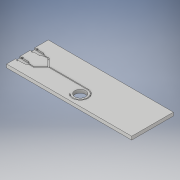
# Autodesk Inventor part: Reactor torus
Saved by Autodesk Inventor 2018 (Build 220112000, 112)
## iProperties
Created: 2018-09-03
Part Number: Reactor torus
Material: Generic
Document SubType Name: Modeling
Designer: mj.noguera10
Density: 1 g/cm^3
Appearance: Default
Author: mj.noguera10
Autodesk Inventor part; units mm, degrees
ref_plane "YZ Plane" through (0, 0, 0) normal (1, 0, 0) x (0, 1, 0)
ref_plane "XZ Plane" through (0, 0, 0) normal (0, 1, 0) x (-1, 0, 0)
ref_plane "XY Plane" through (0, 0, 0) normal (0, 0, 1) x (1, 0, 0)
sketch "Sketch1" plane through (0, 0, 0) normal (0, 1, 0) x (-1, 0, 0)
  line L0 (0, 0) -> (-75, 0)
  line L1 (-75, 0) -> (-75, -25)
  line L2 (-75, -25) -> (0, -25)
  line L3 (0, -25) -> (0, 0)
  dimension "d0" = 75
  dimension "d1" = 25
  constraints: 8 end point, 2 parallel, 1 horizontal, 1 perpendicular
  measures "d0" distance of L2.end L1.end
  measures "d1" distance of L1.end L0.end
extrude "Extrusion1" add sketch "Sketch1" along normal blind 2
sketch "Sketch6" plane through (0, 0, 0) normal (0, -1, 0) x (1, 0, 0)
  circle A0 centre (37.5, -6.6366) radius 3.25
  line L0 (34.4948, -3.6314) -> (34.1412, -3.2779)
  arc A1 (40.5052, -9.6418) -> (34.4948, -3.6314) centre (37.5, -6.6366) ccw
  arc A2 (40.8588, -9.9954) -> (34.1412, -3.2779) centre (37.5, -6.6366) ccw
  line L1 (40.5052, -9.6418) -> (40.8588, -9.9954)
  point P0 (0, 0)
  dimension "d119" = 6.5
  constraints: 4 end point, 4 point on circle, 3 centre point, 1 coincident
  measures "d119" diameter of A0
sketch "Sketch7" plane through (0, 0, 0) normal (0, -1, 0) x (1, 0, 0)
  line L0 (33.6052, -25) -> (33.6052, -24)
  line L1 (32.6052, -17.7) -> (33.6052, -19.7)
  line L2 (32.1052, -17.7) -> (31.1052, -19.7)
  line L3 (34.1052, -23.2) -> (33.6052, -23.2)
  line L4 (34.1052, -24) -> (34.1052, -23.2)
  line L5 (33.6052, -24) -> (34.1052, -24)
  line L6 (30.6052, -24) -> (31.1052, -24)
  line L7 (30.6052, -23.2) -> (30.6052, -24)
  line L8 (33.6052, -25) -> (31.1052, -25)
  line L9 (31.1052, -24) -> (31.1052, -25)
  line L10 (31.1052, -23.2) -> (30.6052, -23.2)
  arc A0 (34.4948, -3.6314) -> (37.1052, -10.8682) centre (37.5, -6.6366) ccw
  line L11 (32.1052, -17.7) -> (32.1052, -16.4929)
  line L12 (32.6052, -17.7) -> (32.6052, -16.7)
  line L13 (36.6052, -11.9929) -> (32.1052, -16.4929)
  line L14 (32.6052, -16.7) -> (36.8552, -12.45)
  line L15 (36.6052, -11.9929) -> (36.6052, -11.3016)
  line L16 (37.1052, -11.9929) -> (37.1052, -10.8682)
  line L17 (40.9978, -17.7) -> (40.9978, -16.5926)
  line L18 (41.4978, -17.7) -> (41.4978, -16.3855)
  line L19 (40.9978, -16.5926) -> (36.8552, -12.45)
  line L20 (37.1052, -11.9929) -> (41.4978, -16.3855)
  line L21 (40.9978, -17.7) -> (39.9978, -19.7)
  line L22 (41.4978, -17.7) -> (42.4978, -19.7)
  line L23 (39.9978, -19.7) -> (39.9978, -23.2)
  line L24 (42.4978, -23.2) -> (42.4978, -19.7)
  line L25 (39.9978, -23.2) -> (39.4978, -23.2)
  line L26 (42.9978, -23.2) -> (42.4978, -23.2)
  line L27 (39.4978, -23.2) -> (39.4978, -24)
  line L28 (39.4978, -24) -> (39.9978, -24)
  line L29 (42.9978, -24) -> (42.9978, -23.2)
  line L30 (42.4978, -24) -> (42.9978, -24)
  line L31 (39.9978, -24) -> (39.9978, -25)
  line L32 (42.4978, -25) -> (42.4978, -24)
  line L33 (42.4978, -25) -> (39.9978, -25)
  arc A1 (34.1412, -3.2779) -> (36.6052, -11.3016) centre (37.5, -6.6366) ccw
  line L34 (34.4948, -3.6314) -> (34.1412, -3.2779)
  line L35 (31.1052, -19.7) -> (31.1052, -23.2)
  line L36 (33.6052, -19.7) -> (33.6052, -23.2)
  point P0 (0, 0)
  point P1 (0, 0)
  constraints: 74 end point, 4 point on circle, 2 centre point, 2 point on line, 2 vertical, 1 coincident
extrude "Extrusion2" cut sketch "Sketch7" against normal blind 0.9
extrude "Extrusion3" cut sketch "Sketch6" against normal blind 2
sketch "Sketch8" plane through (0, 2, 0) normal (0, 1, 0) x (1, 0, 0)
  arc A0 (40.5052, 9.6418) -> (37.5, 10.8866) centre (37.5, 6.6366) ccw
  line L0 (14.1405, 10.8866) -> (37.5, 10.8866)
  line L1 (14.1405, 11.3866) -> (37.5, 11.3866)
  line L2 (40.5052, 9.6418) -> (40.8588, 9.9954)
  arc A1 (40.8588, 9.9954) -> (37.5, 11.3866) centre (37.5, 6.6366) ccw
  line L3 (14.1405, 11.3866) -> (14.1405, 10.8866)
  line L4 (37.5, 6.6366) -> (37.5, 10.8866)
  point P0 (0, 0)
  dimension "d104" = 3.3588
  dimension "d105" = 3.3588
  constraints: 10 end point, 4 point on circle, 2 centre point, 2 horizontal, 2 vertical, 1 coincident
  measures "d104" horizontal distance of L2.end A0.centre
  measures "d105" horizontal distance of L2.end A0.centre
extrude "Extrusion4" cut sketch "Sketch8" against normal blind 0.9
sketch "Sketch9" plane through (0, 2, 0) normal (0, 1, 0) x (1, 0, 0)
  line L0 (7.3, 15.2792) -> (9.5408, 15.2792)
  line L1 (7.3, 6.8866) -> (9.4334, 6.8866)
  line L2 (7.3, 6.3866) -> (9.6405, 6.3866)
  line L3 (7.3, 15.7792) -> (9.7479, 15.7792)
  line L4 (9.4334, 6.8866) -> (13.6834, 11.1366)
  line L5 (9.5408, 15.2792) -> (13.6834, 11.1366)
  line L6 (14.1405, 10.8866) -> (9.6405, 6.3866)
  line L7 (14.1405, 11.3866) -> (9.7479, 15.7792)
  line L8 (14.1405, 11.3866) -> (14.1405, 10.8866)
  line L9 (7.3, 15.7792) -> (7.3, 15.2792)
  line L10 (7.3, 6.8866) -> (7.3, 6.3866)
  line L11 (37.5, 10.8866) -> (14.1405, 10.8866) projected
  line L12 (14.1405, 11.3866) -> (37.5, 11.3866) projected
  arc A0 (40.5052, 9.6418) -> (37.5, 10.8866) centre (37.5, 6.6366) ccw projected
  arc A1 (34.1412, 3.2779) -> (37.5, 11.3866) centre (37.5, 6.6366) ccw projected
  line L13 (40.8625, 9.9917) -> (38.649, 9.9917)
  point P0 (0, 0)
  dimension "d102" = 3.355
  dimension "d103" = 3.3625
  constraints: 24 end point, 5 horizontal, 2 vertical, 1 perpendicular, 1 point on circle
  measures "d102" vertical distance of L13.start A0.centre
  measures "d103" horizontal distance of L13.start A1.centre
extrude "Extrusion5" cut sketch "Sketch9" against normal blind 0.9 contours L9 L3 L7 L8 L6 L2 L10 L1 L4 L5 L0
sketch "Sketch10" plane through (0, 2, 0) normal (0, 1, 0) x (1, 0, 0)
  line L0 (0, 7.8866) -> (0, 5.3866)
  line L1 (0, 7.8866) -> (1, 7.8866)
  line L2 (1, 5.3866) -> (0, 5.3866)
  line L3 (1, 8.3866) -> (1.8, 8.3866)
  line L4 (1.8, 4.8866) -> (1, 4.8866)
  line L5 (1.8, 5.3866) -> (1.8, 4.8866)
  line L6 (1, 4.8866) -> (1, 5.3866)
  line L7 (1, 7.8866) -> (1, 8.3866)
  line L8 (1.8, 8.3866) -> (1.8, 7.8866)
  line L9 (0, 16.7792) -> (0, 14.2792)
  line L10 (0, 16.7792) -> (1, 16.7792)
  line L11 (1, 14.2792) -> (0, 14.2792)
  line L12 (1, 17.2792) -> (1.8, 17.2792)
  line L13 (1.8, 13.7792) -> (1, 13.7792)
  line L14 (1.8, 14.2792) -> (1.8, 13.7792)
  line L15 (1, 13.7792) -> (1, 14.2792)
  line L16 (5.3, 14.2792) -> (1.8, 14.2792)
  line L17 (1, 16.7792) -> (1, 17.2792)
  line L18 (1.8, 17.2792) -> (1.8, 16.7792)
  line L19 (1.8, 16.7792) -> (5.3, 16.7792)
  line L20 (1.8553, 7.8866) -> (5.3, 7.8866)
  line L21 (1.8, 5.3866) -> (5.3, 5.3866)
  line L22 (7.3, 15.2792) -> (7.3, 15.7792) projected
  line L23 (5.3, 16.7792) -> (7.3, 15.7792)
  line L24 (7.3, 15.7792) -> (7.3, 15.2792)
  line L25 (7.3, 15.2792) -> (5.3, 14.2792)
  line L26 (5.3, 7.8866) -> (7.3, 6.903)
  line L27 (7.3, 6.3866) -> (7.3, 6.8866) projected
  line L28 (7.3, 6.903) -> (7.3, 6.3866)
  line L29 (7.3, 6.3866) -> (5.3, 5.3866)
  point P0 (0, 0)
  dimension "d110" = 5.3
  dimension "d111" = 0.8
  dimension "d112" = 3.5
  dimension "d113" = 1
  dimension "d114" = 2.5
  dimension "d115" = 3.5
  dimension "d116" = 0.5
  dimension "d117" = 0.5
  dimension "d118" = 2.5
  constraints: 56 end point, 13 parallel, 7 horizontal, 4 perpendicular, 2 collinear, 2 point on line
  measures "d110" distance of L9.end L16.start
  measures "d111" distance of L12.start L12.end
  measures "d112" distance of L19.end L18.end
  measures "d113" distance of L9.start L10.end
  measures "d114" distance of L9.start L9.end
  measures "d115" distance of L12.end L13.start
  measures "d116" distance of L11.start L13.end
  measures "d117" distance of L12.start L10.end
  measures "d118" distance from line of L19 L16.start
extrude "Extrusion6" cut sketch "Sketch10" against normal blind 0.9
sketch "Sketch11" plane through (0, 2, 0) normal (0, 1, 0) x (1, 0, 0)
  line L0 (0, 7.8866) -> (0, 5.3866)
  line L1 (0, 7.8866) -> (1, 7.8866)
  line L2 (1, 5.3866) -> (0, 5.3866)
  line L3 (1, 8.3866) -> (1.8, 8.3866)
  line L4 (1.8, 4.8866) -> (1, 4.8866)
  line L5 (1.8, 5.3866) -> (1.8, 4.8866)
  line L6 (1, 4.8866) -> (1, 5.3866)
  line L7 (1, 7.8866) -> (1, 8.3866)
  line L8 (1.8, 8.3866) -> (1.8, 7.8866)
  line L9 (1.8, 5.3866) -> (5.3, 5.3866)
  line L10 (5.3, 7.8866) -> (7.3, 6.8866)
  line L11 (7.3, 6.8866) -> (7.3, 6.3865)
  line L12 (7.3, 6.3865) -> (5.3, 5.3866)
  line L13 (1.8, 7.8866) -> (5.3, 7.8866)
  point P0 (0, 0)
  dimension "d82" = 2
  dimension "d83" = 0.9999
  constraints: 28 end point, 6 parallel, 4 horizontal, 2 perpendicular, 1 point on line
  measures "d82" horizontal distance of L9.end L11.end
  measures "d83" vertical distance of L9.end L11.end
extrude "Extrusion7" cut sketch "Sketch11" against normal blind 0.9
body "Solid1"
